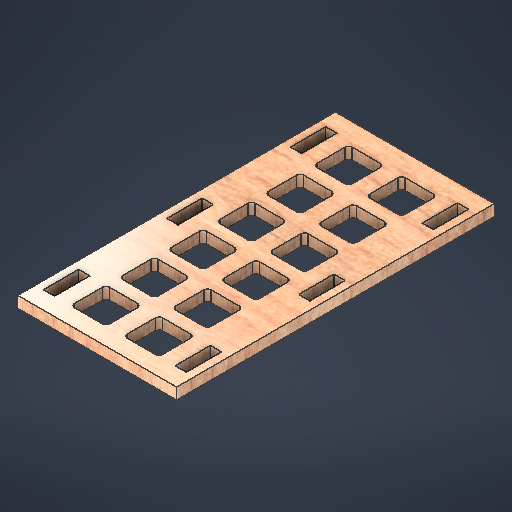
# Autodesk Inventor part: Roof Skiba
Saved by Autodesk Inventor 2027.1 (Build 311270010, 270A)
## iProperties
Created: 2025-11-09
Part Number: Roof Skiba
Material: Generic
Document SubType Name: Modeling
Designer: Nick
Density: 1 g/cm^3
Appearance: Birch - Natural Polished
Mass: 67.8129 g
Surface Area: 326.296 cm^2
Volume: 67.8129 cm^3
Author: Nick
Autodesk Inventor part; units mm, degrees
ref_plane "YZ Plane" through (0, 0, 0) normal (1, 0, 0) x (0, 1, 0)
ref_plane "XZ Plane" through (0, 0, 0) normal (0, 1, 0) x (-1, 0, 0)
ref_plane "XY Plane" through (0, 0, 0) normal (0, 0, 1) x (1, 0, 0)
sketch "Sketch1" plane through (0, 0, 0) normal (0, 1, 0) x (-1, 0, 0)
  line L0 (0, 0) -> (90, 0)
  line L1 (90, 0) -> (90, -180)
  line L2 (90, -180) -> (0, -180)
  line L3 (0, -180) -> (0, 0)
  line L4 (0, 0) -> (4.5, 0)
  line L5 (4.5, 0) -> (4.5, -10) construction
  line L6 (4.5, -10) -> (0, -10) construction
  line L7 (0, -10) -> (0, 0)
  line L8 (4.5, -10) -> (10.85, -10)
  line L9 (10.85, -10) -> (10.85, -30)
  line L10 (10.85, -30) -> (4.5, -30)
  line L11 (4.5, -30) -> (4.5, -10)
  line L12 (4.5, -80) -> (10.85, -80)
  line L13 (10.85, -80) -> (10.85, -100)
  line L14 (10.85, -100) -> (4.5, -100)
  line L15 (4.5, -100) -> (4.5, -80)
  line L16 (4.5, -150) -> (10.85, -150)
  line L17 (10.85, -150) -> (10.85, -170)
  line L18 (10.85, -170) -> (4.5, -170)
  line L19 (4.5, -170) -> (4.5, -150)
  line L20 (45, 0) -> (45, -180) construction
  line L21 (85.5, -10) -> (79.15, -10)
  line L22 (79.15, -10) -> (79.15, -30)
  line L23 (79.15, -30) -> (85.5, -30)
  line L24 (85.5, -30) -> (85.5, -10)
  line L25 (85.5, -80) -> (79.15, -80)
  line L26 (79.15, -80) -> (79.15, -100)
  line L27 (79.15, -100) -> (85.5, -100)
  line L28 (85.5, -100) -> (85.5, -80)
  line L29 (85.5, -150) -> (79.15, -150)
  line L30 (79.15, -150) -> (79.15, -170)
  line L31 (79.15, -170) -> (85.5, -170)
  line L32 (85.5, -170) -> (85.5, -150)
  dimension "d0" = 90
  dimension "d1" = 180
  dimension "d2" = 4.5
  dimension "d3" = 10
  dimension "d4" = 6.35
  dimension "d5" = 20
  dimension "d8" = 70
  constraints: 66 end point, 12 symmetric about line, 6 parallel, 3 horizontal, 3 perpendicular, 2 midpoint, 1 vertical, 16 other
  measures "d0" distance of L1.end L2.end
  measures "d1" distance of L0.end L1.end
  measures "d2" distance of L5.end L6.end
  measures "d3" distance of L4.end L5.end
  measures "d4" distance of L9.end L10.end
  measures "d5" distance of L8.end L9.end
  measures "d8" distance of L5.end L12.start
extrude "Extrusion1" add sketch "Sketch1" along normal blind 6.35
sketch "Sketch2" plane through (0, 6.35, 0) normal (0, 1, 0) x (1, 0, 0)
  line L0 (-90, 180) -> (-90, 0) construction
  line L1 (-90, 0) -> (-70, 0) construction
  line L2 (-70, 0) -> (-70, 10) construction
  line L3 (-70, 10) -> (-90, 10) construction
  line L4 (-90, 10) -> (-90, 0) construction
  line L5 (-68, 10) -> (-52, 10)
  line L6 (-50, 12) -> (-50, 28)
  line L7 (-52, 30) -> (-68, 30)
  line L8 (-70, 28) -> (-70, 12)
  arc A0 (-68, 30) -> (-70, 28) centre (-68, 28) ccw
  arc A1 (-52, 10) -> (-50, 12) centre (-52, 12) ccw
  arc A2 (-50, 28) -> (-52, 30) centre (-52, 28) ccw
  arc A3 (-70, 12) -> (-68, 10) centre (-68, 12) ccw
  arc A4 (-70, 39.5) -> (-68, 37.5) centre (-68, 39.5) ccw
  arc A5 (-52, 37.5) -> (-50, 39.5) centre (-52, 39.5) ccw
  line L9 (-70, 55.5) -> (-70, 39.5)
  line L10 (-52, 57.5) -> (-68, 57.5)
  arc A6 (-68, 57.5) -> (-70, 55.5) centre (-68, 55.5) ccw
  arc A7 (-50, 55.5) -> (-52, 57.5) centre (-52, 55.5) ccw
  line L11 (-50, 39.5) -> (-50, 55.5)
  line L12 (-68, 37.5) -> (-52, 37.5)
  arc A8 (-70, 67) -> (-68, 65) centre (-68, 67) ccw
  arc A9 (-52, 65) -> (-50, 67) centre (-52, 67) ccw
  line L13 (-70, 83) -> (-70, 67)
  line L14 (-52, 85) -> (-68, 85)
  arc A10 (-68, 85) -> (-70, 83) centre (-68, 83) ccw
  arc A11 (-50, 83) -> (-52, 85) centre (-52, 83) ccw
  line L15 (-50, 67) -> (-50, 83)
  line L16 (-68, 65) -> (-52, 65)
  arc A12 (-70, 94.5) -> (-68, 92.5) centre (-68, 94.5) ccw
  arc A13 (-52, 92.5) -> (-50, 94.5) centre (-52, 94.5) ccw
  line L17 (-70, 110.5) -> (-70, 94.5)
  line L18 (-52, 112.5) -> (-68, 112.5)
  arc A14 (-68, 112.5) -> (-70, 110.5) centre (-68, 110.5) ccw
  arc A15 (-50, 110.5) -> (-52, 112.5) centre (-52, 110.5) ccw
  line L19 (-50, 94.5) -> (-50, 110.5)
  line L20 (-68, 92.5) -> (-52, 92.5)
  arc A16 (-40, 12) -> (-38, 10) centre (-38, 12) ccw
  arc A17 (-22, 10) -> (-20, 12) centre (-22, 12) ccw
  line L21 (-40, 28) -> (-40, 12)
  line L22 (-22, 30) -> (-38, 30)
  arc A18 (-38, 30) -> (-40, 28) centre (-38, 28) ccw
  arc A19 (-20, 28) -> (-22, 30) centre (-22, 28) ccw
  line L23 (-20, 12) -> (-20, 28)
  line L24 (-38, 10) -> (-22, 10)
  arc A20 (-40, 39.5) -> (-38, 37.5) centre (-38, 39.5) ccw
  arc A21 (-22, 37.5) -> (-20, 39.5) centre (-22, 39.5) ccw
  line L25 (-40, 55.5) -> (-40, 39.5)
  line L26 (-22, 57.5) -> (-38, 57.5)
  arc A22 (-38, 57.5) -> (-40, 55.5) centre (-38, 55.5) ccw
  arc A23 (-20, 55.5) -> (-22, 57.5) centre (-22, 55.5) ccw
  line L27 (-20, 39.5) -> (-20, 55.5)
  line L28 (-38, 37.5) -> (-22, 37.5)
  arc A24 (-40, 67) -> (-38, 65) centre (-38, 67) ccw
  arc A25 (-22, 65) -> (-20, 67) centre (-22, 67) ccw
  line L29 (-40, 83) -> (-40, 67)
  line L30 (-22, 85) -> (-38, 85)
  arc A26 (-38, 85) -> (-40, 83) centre (-38, 83) ccw
  arc A27 (-20, 83) -> (-22, 85) centre (-22, 83) ccw
  line L31 (-20, 67) -> (-20, 83)
  line L32 (-38, 65) -> (-22, 65)
  arc A28 (-40, 94.5) -> (-38, 92.5) centre (-38, 94.5) ccw
  arc A29 (-22, 92.5) -> (-20, 94.5) centre (-22, 94.5) ccw
  line L33 (-40, 110.5) -> (-40, 94.5)
  line L34 (-22, 112.5) -> (-38, 112.5)
  arc A30 (-38, 112.5) -> (-40, 110.5) centre (-38, 110.5) ccw
  arc A31 (-20, 110.5) -> (-22, 112.5) centre (-22, 110.5) ccw
  line L35 (-20, 94.5) -> (-20, 110.5)
  line L36 (-38, 92.5) -> (-22, 92.5)
  arc A32 (-70, 122) -> (-68, 120) centre (-68, 122) ccw
  arc A33 (-52, 120) -> (-50, 122) centre (-52, 122) ccw
  line L37 (-70, 138) -> (-70, 122)
  line L38 (-52, 140) -> (-68, 140)
  arc A34 (-68, 140) -> (-70, 138) centre (-68, 138) ccw
  arc A35 (-50, 138) -> (-52, 140) centre (-52, 138) ccw
  line L39 (-50, 122) -> (-50, 138)
  line L40 (-68, 120) -> (-52, 120)
  arc A36 (-40, 122) -> (-38, 120) centre (-38, 122) ccw
  arc A37 (-22, 120) -> (-20, 122) centre (-22, 122) ccw
  line L41 (-40, 138) -> (-40, 122)
  line L42 (-22, 140) -> (-38, 140)
  arc A38 (-38, 140) -> (-40, 138) centre (-38, 138) ccw
  arc A39 (-20, 138) -> (-22, 140) centre (-22, 138) ccw
  line L43 (-20, 122) -> (-20, 138)
  line L44 (-38, 120) -> (-22, 120)
  arc A40 (-70, 149.5) -> (-68, 147.5) centre (-68, 149.5) ccw
  arc A41 (-52, 147.5) -> (-50, 149.5) centre (-52, 149.5) ccw
  line L45 (-70, 165.5) -> (-70, 149.5)
  line L46 (-52, 167.5) -> (-68, 167.5)
  arc A42 (-68, 167.5) -> (-70, 165.5) centre (-68, 165.5) ccw
  arc A43 (-50, 165.5) -> (-52, 167.5) centre (-52, 165.5) ccw
  line L47 (-50, 149.5) -> (-50, 165.5)
  line L48 (-68, 147.5) -> (-52, 147.5)
  arc A44 (-40, 149.5) -> (-38, 147.5) centre (-38, 149.5) ccw
  arc A45 (-22, 147.5) -> (-20, 149.5) centre (-22, 149.5) ccw
  line L49 (-40, 165.5) -> (-40, 149.5)
  line L50 (-22, 167.5) -> (-38, 167.5)
  arc A46 (-38, 167.5) -> (-40, 165.5) centre (-38, 165.5) ccw
  arc A47 (-20, 165.5) -> (-22, 167.5) centre (-22, 165.5) ccw
  line L51 (-20, 149.5) -> (-20, 165.5)
  line L52 (-38, 147.5) -> (-22, 147.5)
  point P0 (0, 0)
  point P1 (-50, 30)
  point P2 (-50, 10)
  point P3 (-70, 30)
  point P4 (-50, 37.5)
  point P5 (-70, 57.5)
  point P6 (-70, 37.5)
  point P7 (-50, 57.5)
  point P8 (-50, 65)
  point P9 (-70, 85)
  point P10 (-70, 65)
  point P11 (-50, 85)
  point P12 (-50, 92.5)
  point P13 (-70, 112.5)
  point P14 (-70, 92.5)
  point P15 (-50, 112.5)
  point P16 (-20, 10)
  point P17 (-40, 30)
  point P18 (-40, 10)
  point P19 (-20, 30)
  point P20 (-20, 37.5)
  point P21 (-40, 57.5)
  point P22 (-40, 37.5)
  point P23 (-20, 57.5)
  point P24 (-20, 65)
  point P25 (-40, 85)
  point P26 (-40, 65)
  point P27 (-20, 85)
  point P28 (-20, 92.5)
  point P29 (-40, 112.5)
  point P30 (-40, 92.5)
  point P31 (-20, 112.5)
  point P32 (-50, 120)
  point P33 (-70, 140)
  point P34 (-70, 120)
  point P35 (-50, 140)
  point P36 (-20, 120)
  point P37 (-40, 140)
  point P38 (-40, 120)
  point P39 (-20, 140)
  point P40 (-50, 147.5)
  point P41 (-70, 167.5)
  point P42 (-70, 147.5)
  point P43 (-50, 167.5)
  point P44 (-20, 147.5)
  point P45 (-40, 167.5)
  point P46 (-40, 147.5)
  point P47 (-20, 167.5)
  dimension "d15" = 20
  dimension "d16" = 10
  dimension "d17" = 20
  dimension "d18" = 20
  dimension "d19" = 2
  dimension "d22" = 27.5
  dimension "d25" = 30
  constraints: 104 end point, 96 point on circle, 96 point on line, 48 centre point, 8 tangent, 4 parallel, 3 equal radius, 3 horizontal, 2 perpendicular, 1 vertical, 264 other
  measures "d15" distance of L3.end L2.end
  measures "d16" distance of L2.end L1.end
  measures "d17" distance of point (-70, 30) point (-50, 30)
  measures "d18" distance of point (-50, 30) point (-50, 10)
  measures "d19" radius of A0
  measures "d22" distance of L8.end L9.end
  measures "d25" distance of L8.end L21.end
extrude "Extrusion2" cut sketch "Sketch2" against normal blind 6.35
body "Solid1"
